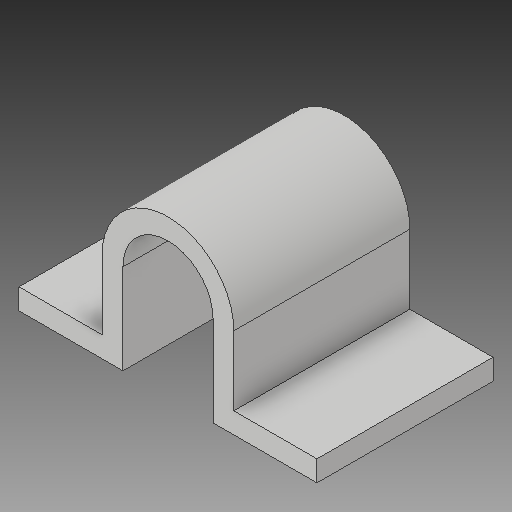
# Autodesk Inventor part: SADDLE_CPY
Saved by Autodesk Inventor 2018 (Build 220112000, 112)
## iProperties
Created: 2021-03-02
Part Number: SADDLE_CPY
Material: Generic
Document SubType Name: Modeling
Designer: Default
Density: 1 g/cm^3
Appearance: Default
Author: Default
Autodesk Inventor part; units mm, degrees
ref_plane "YZ Plane" through (0, 0, 0) normal (1, 0, 0) x (0, 1, 0)
ref_plane "XZ Plane" through (0, 0, 0) normal (0, 1, 0) x (-1, 0, 0)
ref_plane "XY Plane" through (0, 0, 0) normal (0, 0, 1) x (1, 0, 0)
sketch "Sketch1" plane through (0, 0, 0) normal (0, 0, 1) x (1, 0, 0)
  line L0 (0, 0) -> (0, 3)
  line L1 (0, 3) -> (12, 3)
  line L2 (0, 0) -> (15, 0)
  line L3 (15, 0) -> (15, 13)
  line L4 (12, 3) -> (12, 13)
  line L5 (28, 13) -> (28, 0)
  line L6 (28, 0) -> (43, 0)
  line L7 (43, 0) -> (43, 3)
  line L8 (43, 3) -> (31, 3)
  line L9 (31, 3) -> (31, 13)
  arc A0 (28, 13) -> (15, 13) centre (21.5, 13) ccw
  arc A1 (31, 13) -> (12, 13) centre (21.5, 13) ccw
  dimension "d10" = 3
  constraints: 20 end point, 5 perpendicular, 4 point on circle, 2 centre point, 2 vertical, 1 coincident, 1 horizontal, 1 parallel
  measures "d10" distance between parallel lines of L2 L1
extrude "Extrusion1" add sketch "Sketch1" along normal blind 25.4
body "Solid1"
